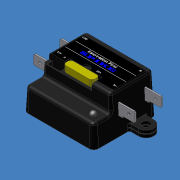
# Autodesk Inventor part: spike_relay
Saved by Autodesk Inventor 2012 (Build 160160000, 160)
## iProperties
Company: Team 801
Created: 2006-05-31
Part Number: spike_relay
Document SubType Name: Modeling
Designer: Jeffrey M
Catalog Web Link: www.team801.org
Density: 1 g/cm^3
Material: Default
Author: Jeffrey M
Autodesk Inventor part; units mm, degrees
ref_plane "YZ Plane" through (0, 0, 0) normal (1, 0, 0) x (0, 1, 0)
ref_plane "XZ Plane" through (0, 0, 0) normal (0, 1, 0) x (-1, 0, 0)
ref_plane "XY Plane" through (0, 0, 0) normal (0, 0, 1) x (1, 0, 0)
sketch "Sketch1" plane through (0, 0, 0) normal (0, 0, 1) x (1, 0, 0)
  line L0 (-20.1295, 14.8818) -> (20.1295, 14.8818)
  line L1 (23.3045, 11.7068) -> (23.3045, -23.5992)
  line L2 (20.1295, -26.7742) -> (-20.1295, -26.7742)
  line L3 (-23.3045, -23.5992) -> (-23.3045, 11.7068)
  arc A0 (-20.1295, 14.8818) -> (-23.3045, 11.7068) centre (-20.1295, 11.7068) ccw
  arc A1 (-23.3045, -23.5992) -> (-20.1295, -26.7742) centre (-20.1295, -23.5992) ccw
  arc A2 (20.1295, -26.7742) -> (23.3045, -23.5992) centre (20.1295, -23.5992) ccw
  arc A3 (23.3045, 11.7068) -> (20.1295, 14.8818) centre (20.1295, 11.7068) ccw
  point P0 (0, 0)
  dimension "d0" = 46.609
  dimension "d1" = 41.656
  dimension "d2" = 3.175
  dimension "d20" = 23.3045
  constraints: 8 end point, 8 point on circle, 8 tangent, 4 centre point, 3 equal radius, 2 parallel, 1 horizontal, 1 perpendicular, 1 other
  measures "d0" distance between parallel lines of L1 L3
  measures "d1" distance between parallel lines of L0 L2
  measures "d2" radius of A0
  measures "d20" distance from line of L1 point (0, 0)
extrude "Extrusion1" add sketch "Sketch1" along normal blind 26.035 draft -3
ref_plane "Work Plane1" through (4.6355, 0, 0) normal (1, 0, 0) x (0, 1, 0)
sketch "Sketch2" plane through (4.6355, 0, 0) normal (1, 0, 0) x (0, 1, 0)
  line L0 (14.8818, 0) -> (13.5174, 26.035) projected
  line L1 (11.7068, 26.035) -> (-23.5992, 26.035) projected
  line L2 (11.7068, 26.035) -> (13.5174, 26.035) projected
  line L3 (2.6864, 26.035) -> (14.1164, 26.035)
  line L4 (14.1164, 26.035) -> (14.1164, 14.605)
  line L5 (14.1164, 14.605) -> (2.6864, 14.605)
  line L6 (2.6864, 14.605) -> (2.6864, 26.035)
  dimension "d6" = 11.43
  dimension "d7" = 11.43
  constraints: 8 end point, 2 parallel, 2 point on line, 1 horizontal, 1 perpendicular
  measures "d6" distance of L4.end L5.end
  measures "d7" distance of L5.end L3.start
extrude "Extrusion2" cut sketch "Sketch2" along normal through all both and the other way through all contours L5 L6 L1 L2 L0
sketch "Sketch3" plane through (0, 0, 0) normal (0, 0, -1) x (-1, 0, 0)
  arc A0 (23.3045, 11.7068) -> (20.1295, 14.8818) centre (20.1295, 11.7068) ccw projected
  line L0 (20.1295, 14.8818) -> (-20.1295, 14.8818) projected
  arc A1 (-20.1295, 14.8818) -> (-23.3045, 11.7068) centre (-20.1295, 11.7068) ccw projected
  line L1 (-23.3045, 11.7068) -> (-23.3045, -23.5992) projected
  arc A2 (-23.3045, -23.5992) -> (-20.1295, -26.7742) centre (-20.1295, -23.5992) ccw projected
  line L2 (-20.1295, -26.7742) -> (20.1295, -26.7742) projected
  arc A3 (20.1295, -26.7742) -> (23.3045, -23.5992) centre (20.1295, -23.5992) ccw projected
  line L3 (23.3045, -23.5992) -> (23.3045, 11.7068) projected
  circle A4 centre (-29.2735, -13.6932) radius 2.54
  arc A5 (-29.2735, -8.6132) -> (-29.2735, -18.7732) centre (-29.2735, -13.6932) ccw
  line L4 (-29.2735, -18.7732) -> (-24.5745, -18.7732)
  line L5 (-24.5745, -8.6132) -> (-29.2735, -8.6132)
  line L6 (-29.2735, -11.1532) -> (-29.2735, -16.2332)
  line L7 (-23.3045, -22.5554) -> (-23.3045, -20.0432)
  line L8 (-23.3045, -7.3432) -> (-23.3045, -4.7439)
  arc A6 (-23.3045, -20.0432) -> (-24.5745, -18.7732) centre (-24.5745, -20.0432) ccw
  arc A7 (-24.5745, -8.6132) -> (-23.3045, -7.3432) centre (-24.5745, -7.3432) ccw
  line L9 (18.6955, -25.9441) -> (18.6955, -20.7088)
  point P0 (-23.3045, -8.6132)
  point P1 (-23.3045, -18.7732)
  dimension "d10" = 5.08
  dimension "d11" = 10.16
  dimension "d12" = 5.969
  dimension "d13" = 8.001
  dimension "d14" = 1.27
  constraints: 12 end point, 8 point on circle, 7 point on line, 6 tangent, 4 centre point, 2 parallel, 1 coincident, 1 collinear, 1 equal radius, 1 horizontal, 1 midpoint
  measures "d10" diameter of A4
  measures "d11" diameter of A5
  measures "d12" distance of L4.start point (-23.305, -18.773)
  measures "d13" distance between parallel lines of L2 L4
  measures "d14" radius of A6
extrude "Extrusion3" add sketch "Sketch3" against normal blind 1.905 contours L1 A6 L4 A5 L5 A7
ref_plane "Work Plane2" through (0, 0, 2.413) normal (0, 0, 1) x (1, 0, 0)
sketch "Sketch4" plane through (0, 0, 2.413) normal (0, 0, 1) x (1, 0, 0)
  line L0 (23.3045, -7.3432) -> (23.3045, -20.0432) projected
  arc A0 (24.5745, -18.7732) -> (23.3045, -20.0432) centre (24.5745, -20.0432) ccw projected
  line L1 (29.2735, -18.7732) -> (24.5745, -18.7732) projected
  arc A1 (29.2735, -18.7732) -> (29.2735, -8.6132) centre (29.2735, -13.6932) ccw projected
  line L2 (24.5745, -8.6132) -> (29.2735, -8.6132) projected
  arc A2 (23.3045, -7.3432) -> (24.5745, -8.6132) centre (24.5745, -7.3432) ccw projected
  circle A3 centre (29.2735, -13.6932) radius 2.54 projected
extrude "Extrusion4" add sketch "Sketch4" along normal blind 1.905
ref_plane "Work Plane3" through (0, 0, 0) normal (1, 0, 0) x (0, 1, 0)
mirror "Mirror1" about plane through (0, 0, 0) normal (1, 0, 0) of "Extrusion4", "Extrusion3"
sketch "Sketch5" plane through (0, 0, 26.035) normal (0, 0, 1) x (1, 0, 0)
  line L0 (22.5391, 11.7068) -> (22.5391, 2.6864) projected
  line L1 (-22.5391, 2.6864) -> (-22.5391, 11.7068) projected
  line L2 (22.5391, 2.6864) -> (-9.8459, 2.6864)
  line L3 (-9.8459, 2.6864) -> (-9.8459, -3.6636)
  line L4 (22.5391, -1.1236) -> (22.5391, 2.6864)
  line L5 (11.7441, -3.6636) -> (11.7441, -1.1236)
  line L6 (11.7441, -1.1236) -> (22.5391, -1.1236)
  line L7 (-9.2109, -4.2986) -> (11.1091, -4.2986)
  arc A0 (11.1091, -4.2986) -> (11.7441, -3.6636) centre (11.1091, -3.6636) ccw
  arc A1 (-9.8459, -3.6636) -> (-9.2109, -4.2986) centre (-9.2109, -3.6636) ccw
  point P0 (-9.8459, -4.2986)
  point P1 (11.7441, -4.2986)
  dimension "d22" = 6.985
  dimension "d23" = 21.59
  dimension "d24" = 10.795
  dimension "d25" = 3.81
  dimension "d26" = 0.635
  dimension "d27" = 0.635
  constraints: 12 end point, 4 point on circle, 4 point on line, 4 tangent, 3 parallel, 2 centre point, 2 horizontal, 1 perpendicular
  measures "d22" distance of L2.end point (-9.846, -4.299)
  measures "d23" distance of point (-9.846, -4.299) point (11.744, -4.299)
  measures "d24" distance of L5.end L4.start
  measures "d25" distance of L4.start L0.end
  measures "d26" radius of A0
  measures "d27" radius of A1
extrude "Extrusion5" cut sketch "Sketch5" against normal blind 4.191
sketch "Sketch6" plane through (-22.5391, 2.6864, 14.605) normal (0, 0, 1) x (1, 0, 0)
  line L0 (45.0782, 9.0204) -> (45.0782, 0) projected
  line L1 (0, 0) -> (45.0782, 0) projected
  circle A0 centre (5.9937, 5.7116) radius 1.905
  line L2 (5.9937, 5.7116) -> (5.9937, 3.8066)
  line L3 (6.8381, 7.5478) -> (6.8381, 7.4193)
  line L4 (5.9937, 5.7116) -> (5.9937, 7.6166)
  dimension "d30" = 3.81
  constraints: 6 end point, 3 parallel, 3 point on circle, 1 centre point, 1 perpendicular
  measures "d30" diameter of A0
revolve "Revolution1" add sketch "Sketch6" angle 360 about axis through (-16.5454, 8.398, 14.605) along (0, 1, 0) picked at (5.8417, 4.4601) contours A0 L4 L2
ref_plane "Work Plane4" through (23.3045, 0, 0) normal (1, 0, 0) x (0, 1, 0)
sketch "Sketch7" plane through (23.3045, 0, 0) normal (1, 0, 0) x (0, 1, 0)
  line L0 (-26.7742, 0) -> (-25.4098, 26.035) projected
  line L1 (-1.1236, 21.844) -> (-1.1236, 26.035) projected
  line L2 (-1.1236, 26.035) -> (-23.5992, 26.035) projected
  line L3 (-23.5992, 0) -> (-23.5992, 26.035) projected
  line L4 (-20.0432, 0) -> (-23.5992, 0) projected
  line L5 (-7.3432, 0) -> (-20.0432, 0) projected
  line L6 (11.7068, 0) -> (-7.3432, 0) projected
  line L7 (11.7068, 0) -> (11.7068, 14.605) projected
  line L8 (11.7068, 14.605) -> (2.6864, 14.605) projected
  line L9 (2.6864, 14.605) -> (2.6864, 21.844) projected
  line L10 (2.6864, 21.844) -> (-1.1236, 21.844) projected
  line L11 (-23.5992, 26.035) -> (-25.4098, 26.035) projected
  line L12 (-26.7742, 0) -> (-25.4098, 26.035) projected
  line L13 (-23.5992, 0) -> (-26.7742, 0) projected
  line L14 (-23.5992, 0) -> (-23.5992, 26.035) projected
  line L15 (14.8818, 0) -> (14.1164, 14.605) projected
  line L16 (11.7068, 0) -> (14.8818, 0) projected
  line L17 (-20.4242, 18.9287) -> (-19.5352, 18.9287)
  line L18 (-19.5352, 18.9287) -> (-19.5352, 11.5627)
  line L19 (-19.5352, 11.5627) -> (-20.4242, 11.5627)
  line L20 (-20.4242, 11.5627) -> (-20.4242, 18.9287)
  line L21 (-3.0252, 18.9287) -> (-2.1362, 18.9287)
  line L22 (-2.1362, 18.9287) -> (-2.1362, 11.5627)
  line L23 (-2.1362, 11.5627) -> (-3.0252, 11.5627)
  line L24 (-3.0252, 11.5627) -> (-3.0252, 18.9287)
  dimension "d33" = 0.889
  dimension "d34" = 7.366
  dimension "d35" = 6.35
  dimension "d36" = 0.889
  dimension "d37" = 16.51
  constraints: 16 end point, 4 parallel, 2 horizontal, 2 perpendicular
  measures "d33" distance between parallel lines of L20 L18
  measures "d34" distance of L19.end L17.start
  measures "d35" distance from line of L0.start L20
  measures "d36" distance of L21.start L21.end
  measures "d37" distance between parallel lines of L18 L24
extrude "Extrusion6" add sketch "Sketch7" along normal blind 10.16 contours L17 L18 L19 L20 | L21 L22 L23 L24
sketch "Sketch8" plane through (23.3045, 0, 0) normal (-1, 0, 0) x (0, 0, 1)
  line L0 (18.9287, -20.4242) -> (18.9287, -19.5352) projected
  line L1 (18.9287, -19.5352) -> (11.5627, -19.5352) projected
  line L2 (11.5627, -19.5352) -> (11.5627, -20.4242) projected
  line L3 (11.5627, -20.4242) -> (18.9287, -20.4242) projected
  line L4 (18.9287, -3.0252) -> (18.9287, -2.1362) projected
  line L5 (18.9287, -2.1362) -> (11.5627, -2.1362) projected
  line L6 (11.5627, -2.1362) -> (11.5627, -3.0252) projected
  line L7 (11.5627, -3.0252) -> (18.9287, -3.0252) projected
extrude "Extrusion7" add sketch "Sketch8" against normal up to surface surface through (23.3045, 11.7068, 0) normal (0.9986295, 0, 0.052336)
sketch "Sketch9" plane through (33.4645, -20.4242, 11.5627) normal (0, -1, 0) x (1, 0, 0)
  line L0 (0, 0) -> (0, 7.366) projected
  line L1 (-11.152, 7.366) -> (0, 7.366) projected
  line L2 (0, 0) -> (-10.766, 0) projected
  line L3 (-8.226, 0) -> (-8.226, 1.016)
  line L4 (-8.226, 1.016) -> (-0.635, 1.016)
  circle A0 centre (-4.1272, 4.191) radius 0.9525
  line L5 (-8.226, 7.366) -> (-8.226, 1.016)
  line L6 (-8.226, 1.016) -> (0, 1.016)
  line L7 (0, 1.651) -> (0, 6.731)
  line L8 (-8.226, 1.016) -> (0, 1.016)
  line L9 (0, 1.016) -> (0, 0)
  line L10 (0, 0) -> (-8.226, 0)
  line L11 (-8.226, 0) -> (-8.226, 1.016)
  line L12 (0, 6.731) -> (-0.635, 7.366)
  line L13 (-0.635, 1.016) -> (0, 1.651)
  line L14 (-0.635, 7.366) -> (0, 6.731)
  line L15 (0, 7.366) -> (-0.635, 7.366)
  line L16 (0, 7.366) -> (0, 6.731)
  line L17 (-0.635, 1.016) -> (0, 1.016)
  line L18 (0, 1.016) -> (0, 1.651)
  line L19 (0, 1.651) -> (-0.635, 1.016)
  line L20 (-10.766, 0) -> (-11.152, 7.366) projected
  point P0 (0, 1.016)
  dimension "d42" = 1.905
  dimension "d43" = 2.54
  dimension "d44" = 6.35
  dimension "d46" = 8.226
  dimension "d47" = 4.1272
  dimension "d48" = 0.635
  dimension "d49" = 0.635
  dimension "d50" = 0.635
  dimension "d51" = 0.635
  constraints: 34 end point, 7 point on line, 6 perpendicular, 3 parallel, 2 coincident, 1 centre point, 1 collinear, 1 horizontal
  measures "d42" diameter of A0
  measures "d43" distance from line of point (-10.766, 0) L3
  measures "d44" distance between parallel lines of L1 L4
  measures "d46" distance of L3.end point (0, 1.016)
  measures "d47" distance from line of L0 A0.centre
  measures "d48" distance of L7.end L0.end
  measures "d49" distance of L12.end L0.end
  measures "d50" distance of L4.end L17.end
  measures "d51" distance of L7.start L17.end
extrude "Extrusion8" cut sketch "Sketch9" against normal through all contours L2 L3 L4 L6 L0 | L6 L13 L0 | L12 L1 L0 | A0
mirror "Mirror2" about plane through (0, 0, 0) normal (1, 0, 0) of "Extrusion6", "Extrusion8"
sketch "Sketch10" plane through (-23.3045, -3.0252, 18.9287) normal (1, 0, 0) x (0, 0, -1)
  line L0 (0, 0) -> (0, 0.889) projected
  line L1 (7.366, 0) -> (0, 0) projected
  line L2 (7.366, 0.889) -> (7.366, 0) projected
  line L3 (0, 0.889) -> (7.366, 0.889) projected
  line L4 (0, -17.399) -> (0, -16.51) projected
  line L5 (7.366, -17.399) -> (0, -17.399) projected
  line L6 (7.366, -16.51) -> (7.366, -17.399) projected
  line L7 (0, -16.51) -> (7.366, -16.51) projected
extrude "Extrusion9" add sketch "Sketch10" along normal up to surface surface through (-23.3045, -23.5992, 0) normal (-0.9986295, 0, 0.052336)
sketch "Sketch11" plane through (0, 0, 21.844) normal (0, 0, 1) x (1, 0, 0)
  line L0 (11.7441, -3.6636) -> (11.7441, -1.1236) projected
  line L1 (11.7441, -1.1236) -> (22.1597, -1.1236) projected
  line L2 (19.9991, -1.1236) -> (11.7441, -1.1236)
  line L3 (11.7441, -1.1236) -> (11.7441, 2.0514)
  line L4 (11.7441, 2.0514) -> (19.9991, 2.0514)
  line L5 (19.9991, 2.0514) -> (19.9991, -1.1236)
  dimension "d56" = 3.175
  dimension "d57" = 8.255
  dimension "d58" = 0
  dimension "d60" = 0
  constraints: 8 end point, 2 parallel, 1 horizontal, 1 perpendicular
  measures "d56" distance of L2.end L3.end
  measures "d57" distance of L3.end L4.end
  measures "d58" distance between parallel lines of L1 L2
  measures "d60" distance between parallel lines of L0 L3
extrude "Extrusion10" cut sketch "Sketch11" against normal blind 7.239
sketch "Sketch12" plane through (0, 0, 14.605) normal (0, 0, 1) x (1, 0, 0)
  line L0 (19.9991, 2.0514) -> (11.7441, 2.0514) projected
  line L1 (11.7441, -1.1236) -> (19.9991, -1.1236) projected
  line L2 (12.8285, 1.0989) -> (14.0985, 1.0989)
  line L3 (14.0985, 1.0989) -> (14.0985, -0.1711)
  line L4 (14.0985, -0.1711) -> (12.8285, -0.1711)
  line L5 (12.8285, -0.1711) -> (12.8285, 1.0989)
  line L6 (15.3685, 1.0989) -> (16.6385, 1.0989)
  line L7 (16.6385, 1.0989) -> (16.6385, -0.1711)
  line L8 (16.6385, -0.1711) -> (15.3685, -0.1711)
  line L9 (15.3685, -0.1711) -> (15.3685, 1.0989)
  line L10 (17.9085, 1.0989) -> (19.1785, 1.0989)
  line L11 (19.1785, 1.0989) -> (19.1785, -0.1711)
  line L12 (19.1785, -0.1711) -> (17.9085, -0.1711)
  line L13 (17.9085, -0.1711) -> (17.9085, 1.0989)
  dimension "d63" = 1.27
  dimension "d64" = 1.27
  dimension "d67" = 2.54
  dimension "d72" = 0.9525
  dimension "d73" = 0.9525
  constraints: 24 end point, 2 horizontal, 2 parallel, 1 perpendicular, 16 other
  measures "d63" distance of L2.start L2.end
  measures "d64" distance of L2.end L3.end
  measures "d67" distance of L2.start L6.start
  measures "d72" distance between parallel lines of L0 L2
  measures "d73" distance between parallel lines of L1 L4
extrude "Extrusion11" cut sketch "Sketch12" against normal blind 0.635 draft -40
sketch "Sketch13" plane through (0, 0, 26.035) normal (0, 0, 1) x (1, 0, 0)
  line L0 (11.1091, -4.2986) -> (-9.2109, -4.2986) projected
  arc A0 (-1.5909, -4.2986) -> (3.4891, -4.2986) centre (0.9491, -4.2986) ccw
  dimension "d76" = 5.08
  constraints: 2 point on circle, 2 point on line, 1 centre point, 1 midpoint
  measures "d76" diameter of A0
extrude "Extrusion12" cut sketch "Sketch13" against normal blind 0.889
sketch "Sketch14" plane through (0, 0, 21.844) normal (0, 0, 1) x (1, 0, 0)
  line L0 (8.8549, -3.9966) -> (-6.3851, -3.9966)
  line L1 (-8.2901, -2.0916) -> (-8.2901, -0.8216)
  line L2 (-6.3851, 1.0834) -> (8.8549, 1.0834)
  line L3 (10.7599, -0.8216) -> (10.7599, -2.0916)
  arc A0 (8.8549, -3.9966) -> (10.7599, -2.0916) centre (8.8549, -2.0916) ccw
  arc A1 (10.7599, -0.8216) -> (8.8549, 1.0834) centre (8.8549, -0.8216) ccw
  arc A2 (-6.3851, 1.0834) -> (-8.2901, -0.8216) centre (-6.3851, -0.8216) ccw
  arc A3 (-8.2901, -2.0916) -> (-6.3851, -3.9966) centre (-6.3851, -2.0916) ccw
  point P0 (10.7599, -3.9966)
  point P1 (-8.2901, 1.0834)
  point P2 (10.7599, 1.0834)
  dimension "d79" = 19.05
  dimension "d80" = 5.08
  dimension "d81" = 1.905
  constraints: 8 end point, 8 point on circle, 8 tangent, 6 point on line, 4 centre point, 3 equal radius, 2 parallel, 1 horizontal, 1 perpendicular
  measures "d79" distance of point (-8.29, 1.083) point (10.76, 1.083)
  measures "d80" distance of point (10.76, 1.083) point (10.76, -3.997)
  measures "d81" radius of A0
extrude "Extrusion13" add sketch "Sketch14" along normal up to surface (4.191 mm away)
fillet "Fillet1" radius 1.524 14 edges at (-21.9401, -10.4564, 26.035) (-21.4098, -24.8795, 26.035) (0, -25.4098, 26.035) (21.4098, -24.8795, 26.035) (21.9401, -12.3614, 26.035) (-15.893, 2.6864, 26.035) (0, 2.6864, 14.605) (0, 14.1164, 14.605) (21.8333, 13.4106, 14.605) (22.5391, 7.1966, 14.605) (-21.8333, 13.4106, 14.605) (-22.5391, 7.1966, 14.605) (-22.2396, 2.6864, 20.32) (22.3494, 2.6864, 18.2245)
decal "Decal1"
sketch "Sketch16" plane through (-33.4645, -3.0252, 13.2137) normal (0, -1, 0) x (1, 0, 0)
  circle A0 centre (4.1272, 2.54) radius 0.9525 projected
sketch "Sketch17" plane through (-33.4645, -20.4242, 13.2137) normal (0, -1, 0) x (1, 0, 0)
  circle A0 centre (4.1272, 2.54) radius 0.9525 projected
sketch "Sketch18" plane through (33.4645, -3.0252, 13.2137) normal (0, -1, 0) x (1, 0, 0)
  circle A0 centre (-4.1272, 2.54) radius 0.9525 projected
sketch "Sketch19" plane through (33.4645, -20.4242, 13.2137) normal (0, -1, 0) x (1, 0, 0)
  circle A0 centre (-4.1272, 2.54) radius 0.9525 projected
sketch "Sketch15" plane through (0, 0, 26.035) normal (0, 0, 1) x (1, 0, 0)
  line L0 (20.752, -22.1482) -> (-21.158, -22.1482) construction
  line L1 (-21.158, -22.1482) -> (-21.158, -0.7758) construction
  line L2 (-21.158, -0.7758) -> (20.752, -0.7758) construction
  line L3 (20.752, -0.7758) -> (20.752, -22.1482) construction
  dimension "d86" = 41.91
  constraints: 2 other
  measures "d86" distance of L0.start L0.end
equation "\"d49\" = d48"
equation "\"d50\" = d48"
equation "\"d51\" = d50"
body "Solid1"
